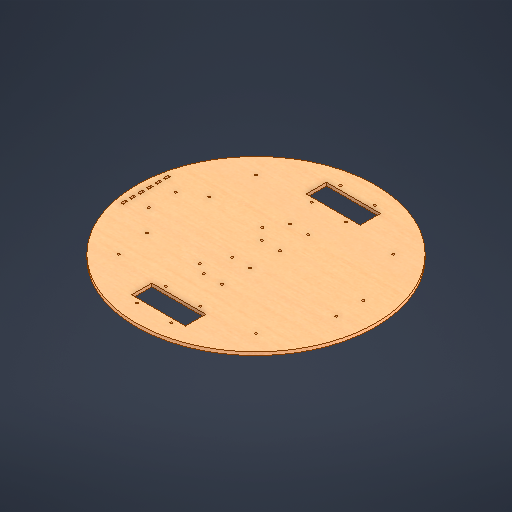
# Autodesk Inventor part: layer1
Saved by Autodesk Inventor 2026 (Build 300175050, 175E)
## iProperties
Created: 2025-06-04
Part Number: layer1
Material: Generic
Document SubType Name: Modeling
Designer: satom
Density: 1 g/cm^3
Appearance: Cherry - Natural Low Gloss
Author: satom
Autodesk Inventor part; units mm, degrees
ref_plane "YZ Plane" through (0, 0, 0) normal (1, 0, 0) x (0, 1, 0)
ref_plane "XZ Plane" through (0, 0, 0) normal (0, 1, 0) x (-1, 0, 0)
ref_plane "XY Plane" through (0, 0, 0) normal (0, 0, 1) x (1, 0, 0)
sketch "Sketch1" plane through (0, 0, 0) normal (0, 1, 0) x (-1, 0, 0)
  circle A0 centre (0, 0) radius 177
  dimension "d0" = 354
  constraints: 1 centre point, 1 coincident
  measures "d0" diameter of A0
extrude "Extrusion1" add sketch "Sketch1" along normal blind 4.7625
sketch "Sketch2" plane through (0, 4.7625, 0) normal (0, 1, 0) x (1, 0, 0)
  circle A0 centre (101.6, -101.6) radius 1.7
  circle A1 centre (101.6, 101.6) radius 1.7
  circle A2 centre (-101.6, 101.6) radius 1.7
  circle A3 centre (-101.6, -101.6) radius 1.7
  circle A4 centre (0, 0) radius 177 projected
  dimension "d3" = 3.4
  dimension "d4" = 3.4
  dimension "d5" = 3.4
  dimension "d6" = 3.4
  dimension "d14" = 101.6
  dimension "d15" = 101.6
  dimension "d16" = 101.6
  dimension "d17" = 101.6
  dimension "d18" = 101.6
  dimension "d19" = 101.6
  dimension "d20" = 101.6
  dimension "d21" = 101.6
  constraints: 4 centre point
  measures "d3" diameter of A3
  measures "d4" diameter of A2
  measures "d5" diameter of A0
  measures "d6" diameter of A1
  measures "d14" horizontal distance of point (0, 0) A3.centre
  measures "d15" horizontal distance of point (0, 0) A3.centre
  measures "d16" horizontal distance of point (0, 0) A0.centre
  measures "d17" horizontal distance of point (0, 0) A0.centre
  measures "d18" horizontal distance of point (0, 0) A1.centre
  measures "d19" horizontal distance of point (0, 0) A1.centre
  measures "d20" horizontal distance of point (0, 0) A2.centre
  measures "d21" horizontal distance of point (0, 0) A2.centre
extrude "Standoff Holes" cut sketch "Sketch2" against normal through all contours A0 | A1 | A2 | A3
sketch "Sketch3" plane through (0, 4.7625, 0) normal (0, 1, 0) x (1, 0, 0)
  line L0 (-40, -144.3) -> (40, -144.3)
  line L1 (40, -144.3) -> (40, -114.3)
  line L2 (40, -114.3) -> (-40, -114.3)
  line L3 (-40, -114.3) -> (-40, -144.3)
  circle A0 centre (-25.4, -107.95) radius 1.7
  circle A1 centre (25.4, -107.95) radius 1.7
  circle A2 centre (25.4, -150.65) radius 1.7
  circle A3 centre (-25.4, -150.65) radius 1.7
  circle A4 centre (0, 0) radius 177 projected
  line L4 (-177, 0) -> (177, 0)
  line L5 (-40, 144.3) -> (40, 144.3)
  line L6 (40, 144.3) -> (40, 114.3)
  line L7 (40, 114.3) -> (-40, 114.3)
  line L8 (-40, 114.3) -> (-40, 144.3)
  circle A5 centre (-25.4, 107.95) radius 1.7
  circle A6 centre (25.4, 107.95) radius 1.7
  circle A7 centre (25.4, 150.65) radius 1.7
  circle A8 centre (-25.4, 150.65) radius 1.7
  point P0 (0, -114.3)
  point P1 (0, 114.3)
  dimension "d25" = 80
  dimension "d26" = 30
  dimension "d28" = 114.3
  dimension "d30" = 40
  dimension "d32" = 3.4
  dimension "d33" = 3.4
  dimension "d34" = 3.4
  dimension "d35" = 3.4
  dimension "d36" = 6.35
  dimension "d37" = 6.35
  dimension "d38" = 6.35
  dimension "d39" = 6.35
  dimension "d40" = 25.4
  dimension "d41" = 25.4
  dimension "d42" = 25.4
  dimension "d43" = 25.4
  dimension "d44" = 228.6
  constraints: 18 end point, 9 symmetric about line, 8 centre point, 2 horizontal, 2 parallel, 2 point on circle, 1 midpoint, 1 perpendicular, 4 other
  measures "d25" distance of L0.start L0.end
  measures "d26" distance of L2.end L0.start
  measures "d28" distance from line of point (0, 0) L2
  measures "d30" distance from line of point (0, 0) L3
  measures "d32" diameter of A0
  measures "d33" diameter of A1
  measures "d34" diameter of A2
  measures "d35" diameter of A3
  measures "d36" distance from line of L2 A0.centre
  measures "d37" distance from line of L2 A1.centre
  measures "d38" distance from line of L0 A2.centre
  measures "d39" distance from line of L0 A3.centre
  measures "d40" horizontal distance of point (0, 0) A3.centre
  measures "d41" horizontal distance of point (0, 0) A2.centre
  measures "d42" horizontal distance of point (0, 0) A1.centre
  measures "d43" horizontal distance of A0.centre point (0, 0)
  measures "d44" diameter of L7 L4
extrude "Wheels" cut sketch "Sketch3" against normal blind 25.4 contours L3 L2 L1 L0 | A0 | A1 | A2 | A3 | L5 L6 L7 L8 | A5 | A6 | A7 | A8
sketch "Sketch4" plane through (0, 4.7625, 0) normal (0, 1, 0) x (1, 0, 0)
  circle A0 centre (13.4493, -63.76) radius 1.7
  circle A1 centre (13.4493, -21.9516) radius 1.7
  circle A2 centre (-13.4493, -63.76) radius 1.7
  circle A3 centre (-13.4493, -21.9516) radius 1.7
  line L0 (-40, -114.3) -> (40, -114.3) projected
  circle A4 centre (0, 0) radius 177 projected
  line L1 (-177, 0) -> (177, 0) construction
  circle A5 centre (13.4493, 63.76) radius 1.7
  circle A6 centre (13.4493, 21.9516) radius 1.7
  circle A7 centre (-13.4493, 63.76) radius 1.7
  circle A8 centre (-13.4493, 21.9516) radius 1.7
  dimension "d47" = 3.4
  dimension "d48" = 3.4
  dimension "d49" = 3.4
  dimension "d50" = 3.4
  dimension "d51" = 26.8986
  dimension "d52" = 26.8986
  dimension "d53" = 41.8084
  dimension "d54" = 41.8084
  dimension "d55" = 13.4493
  dimension "d56" = 13.4493
  dimension "d57" = 50.54
  dimension "d84" = 13.4493
  constraints: 8 centre point, 4 symmetric about line, 2 end point, 2 point on circle, 1 horizontal, 1 midpoint, 4 other
  measures "d47" diameter of A2
  measures "d48" diameter of A3
  measures "d49" diameter of A0
  measures "d50" diameter of A1
  measures "d51" distance of A0.centre A2.centre
  measures "d52" distance of A1.centre A3.centre
  measures "d53" distance of A1.centre A0.centre
  measures "d54" distance of A2.centre A3.centre
  measures "d55" horizontal distance of point (0, 0) A2.centre
  measures "d56" horizontal distance of point (0, 0) A3.centre
  measures "d57" distance from line of L0 A0.centre
  measures "d84" horizontal distance of point (0, 0) A0.centre
extrude "Motor Mount" cut sketch "Sketch4" against normal through all contours A0 | A1 | A2 | A3 | A5 | A6 | A7 | A8
sketch "Sketch5" plane through (0, 4.7625, 0) normal (0, 1, 0) x (1, 0, 0)
  circle A0 centre (-107.95, -53.7) radius 1.7
  circle A1 centre (-107.95, 38.8) radius 1.7
  circle A2 centre (-29.45, 38.8) radius 1.7
  circle A3 centre (-29.45, -53.7) radius 1.7
  point P0 (0, 0)
  dimension "d61" = 3.4
  dimension "d62" = 3.4
  dimension "d63" = 3.4
  dimension "d64" = 3.4
  dimension "d65" = 92.5
  dimension "d66" = 92.5
  dimension "d67" = 78.5
  dimension "d68" = 78.5
  dimension "d69" = 38.8
  dimension "d70" = 38.8
  dimension "d72" = 53.7
  dimension "d73" = 107.95
  constraints: 4 centre point
  measures "d61" diameter of A0
  measures "d62" diameter of A1
  measures "d63" diameter of A2
  measures "d64" diameter of A3
  measures "d65" distance of A1.centre A0.centre
  measures "d66" distance of A3.centre A2.centre
  measures "d67" distance of A3.centre A0.centre
  measures "d68" distance of A2.centre A1.centre
  measures "d69" vertical distance of point (0, 0) A1.centre
  measures "d70" vertical distance of point (0, 0) A2.centre
  measures "d72" vertical distance of point (0, 0) A0.centre
  measures "d73" horizontal distance of point (0, 0) A1.centre
extrude "PCB" cut sketch "Sketch5" against normal blind 25.4
sketch "Sketch6" plane through (0, 4.7625, 0) normal (0, 1, 0) x (1, 0, 0)
  circle A0 centre (138.9, -20) radius 1.7
  circle A1 centre (138.9, 20) radius 1.7
  circle A2 centre (0, 0) radius 177 projected
  line L0 (177, 0) -> (177, 59.2823) construction
  line L1 (0, -177) -> (0, 177) construction
  circle A3 centre (-138.9, -20) radius 1.7
  circle A4 centre (-138.9, 20) radius 1.7
  dimension "d76" = 3.4
  dimension "d77" = 3.4
  dimension "d78" = 40
  dimension "d80" = 20
  dimension "d81" = 38.1
  constraints: 4 centre point, 4 end point, 3 point on circle, 2 symmetric about line, 2 vertical, 1 tangent, 2 other
  measures "d76" diameter of A0
  measures "d77" diameter of A1
  measures "d78" distance of A1.centre A0.centre
  measures "d80" vertical distance of point (0, 0) A0.centre
  measures "d81" distance from line of L0 A0.centre
extrude "Caster" cut sketch "Sketch6" against normal blind 25.4 contours A0 | A1 | A3 | A4
sketch "Sketch7" plane through (0, 4.7625, 0) normal (0, 1, 0) x (1, 0, 0)
  line L0 (-166.0395, -33.995) -> (-162.8645, -33.995)
  line L1 (-162.8645, -33.995) -> (-162.8645, -27.645)
  line L2 (-162.8645, -27.645) -> (-166.0395, -27.645)
  line L3 (-166.0395, -27.645) -> (-166.0395, -33.995)
  line L4 (-162.8645, -21.295) -> (-162.8645, -14.945)
  line L5 (-162.8645, -14.945) -> (-166.0395, -14.945)
  line L6 (-166.0395, -14.945) -> (-166.0395, -21.295)
  line L7 (-166.0395, -21.295) -> (-162.8645, -21.295)
  line L8 (-162.8645, -8.595) -> (-162.8645, -2.245)
  line L9 (-162.8645, -2.245) -> (-166.0395, -2.245)
  line L10 (-166.0395, -2.245) -> (-166.0395, -8.595)
  line L11 (-166.0395, -8.595) -> (-162.8645, -8.595)
  line L12 (-162.8645, 4.105) -> (-162.8645, 10.455)
  line L13 (-162.8645, 10.455) -> (-166.0395, 10.455)
  line L14 (-166.0395, 10.455) -> (-166.0395, 4.105)
  line L15 (-166.0395, 4.105) -> (-162.8645, 4.105)
  line L16 (-162.8645, 16.805) -> (-162.8645, 23.155)
  line L17 (-162.8645, 23.155) -> (-166.0395, 23.155)
  line L18 (-166.0395, 23.155) -> (-166.0395, 16.805)
  line L19 (-166.0395, 16.805) -> (-162.8645, 16.805)
  line L20 (-162.8645, 29.505) -> (-162.8645, 35.855)
  line L21 (-162.8645, 35.855) -> (-166.0395, 35.855)
  line L22 (-166.0395, 35.855) -> (-166.0395, 29.505)
  line L23 (-166.0395, 29.505) -> (-162.8645, 29.505)
  point P0 (0, 0)
  dimension "d85" = 6.35
  dimension "d86" = 3.175
  dimension "d89" = 12.7
  dimension "d94" = 162.8645
  dimension "d95" = 33.995
  constraints: 48 end point, 2 parallel, 1 collinear, 1 horizontal, 1 perpendicular, 1 vertical, 39 other
  measures "d85" distance of L2.end L0.start
  measures "d86" distance of L0.start L0.end
  measures "d89" distance of L0.start L6.end
  measures "d94" distance from line of L1 point (0, 0)
  measures "d95" distance from line of point (0, 0) L0
extrude "Switch" cut sketch "Sketch7" against normal through all
equation "\"d30\" = 0.5 * d25"
equation "\"d52\" = d51"
equation "\"d54\" = d53"
equation "\"d55\" = 0.5 * d51"
equation "\"d56\" = d55"
equation "\"d62\" = d61"
equation "\"d63\" = d61"
equation "\"d64\" = d61"
equation "\"d66\" = d65"
equation "\"d68\" = d67"
equation "\"d70\" = d69"
equation "\"d72\" = d65 - d69"
equation "\"d80\" = 0.5 * d78"
body "Solid1"
